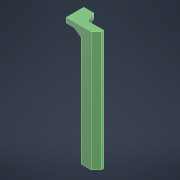
# Autodesk Inventor part: Vertical Beam Prototype
Saved by Autodesk Inventor 2022 (Build 260153000, 153)
## iProperties
Created: 2021-05-30
Part Number: Vertical Beam Prototype
Material: Generic
Document SubType Name: Modeling
Designer: sidsa
Density: 1 g/cm^3
Appearance: Smooth - Dark Forest Green
Author: sidsa
## iProperties of the stored document Vertical Beam Prototype_3DPrint.ipt
Created: 2021-05-30
Part Number: Vertical Beam Prototype_3DPrint
Material: Generic
Document SubType Name: Modeling
Designer: sidsa
Density: 1 g/cm^3
Appearance: Default
Author: sidsa
Autodesk Inventor part; units mm, degrees
ref_plane "YZ Plane" through (0, 0, 0) normal (1, 0, 0) x (0, 1, 0)
ref_plane "XZ Plane" through (0, 0, 0) normal (0, 1, 0) x (-1, 0, 0)
ref_plane "XY Plane" through (0, 0, 0) normal (0, 0, 1) x (1, 0, 0)
sketch "Sketch1" plane through (0, 0, 0) normal (0, 0, 1) x (1, 0, 0)
  line L0 (0, 0) -> (25.4, 0)
  line L1 (25.4, 0) -> (25.4, 152.4)
  line L2 (25.4, 152.4) -> (0, 152.4)
  line L3 (0, 152.4) -> (0, 0)
  line L4 (16.7357, 37.973) -> (20.3652, 31.6865)
  line L5 (20.3652, 31.6865) -> (16.7357, 25.4)
  line L6 (16.7357, 25.4) -> (9.4767, 25.4)
  line L7 (9.4767, 25.4) -> (5.8472, 31.6865)
  line L8 (5.8472, 31.6865) -> (9.4767, 37.973)
  line L9 (9.4767, 37.973) -> (16.7357, 37.973)
  line L10 (12.7, 0) -> (13.1062, 31.6865)
  dimension "d0" = 25.4
  dimension "d1" = 152.4
  dimension "d2" = 12.573
  dimension "d3" = 25.4
  constraints: 22 end point, 3 parallel, 1 horizontal, 1 midpoint, 1 perpendicular, 13 other
  measures "d0" distance of L1.end L2.end
  measures "d1" distance of L0.end L1.end
  measures "d2" distance between parallel lines of L6 L9
  measures "d3" distance between parallel lines of L0 L6
extrude "Extrusion1" add sketch "Sketch1" along normal blind 3.175
sketch "Sketch2" plane through (0, 0, 0) normal (0, 0, -1) x (-1, 0, 0)
  line L0 (-25.4, 0) -> (-25.4, 152.4) projected
  line L1 (0, 0) -> (-25.4, 0) projected
  line L2 (0, 152.4) -> (0, 0) projected
  line L3 (-25.4, 152.4) -> (0, 152.4) projected
  line L4 (-16.7357, 25.4) -> (-9.4767, 25.4) projected
  line L5 (-20.3652, 31.6865) -> (-16.7357, 25.4) projected
  line L6 (-16.7357, 37.973) -> (-20.3652, 31.6865) projected
  line L7 (-9.4767, 37.973) -> (-16.7357, 37.973) projected
  line L8 (-5.8472, 31.6865) -> (-9.4767, 37.973) projected
  line L9 (-9.4767, 25.4) -> (-5.8472, 31.6865) projected
extrude "Extrusion2" add sketch "Sketch2" along normal blind 3.175 and the other way blind 3.175 contours L5 L6 L7 L8 L9 L4
sketch "Sketch3" plane through (0, 0, 3.175) normal (0, 0, 1) x (1, 0, 0)
  line L0 (25.4, 0) -> (25.4, 152.4) projected
  line L1 (25.4, 152.4) -> (0, 152.4) projected
  line L2 (0, 152.4) -> (0, 0) projected
  line L3 (0, 0) -> (25.4, 0) projected
extrude "Extrusion3" add sketch "Sketch3" along normal blind 6.35
chamfer "Chamfer1" distance 6.35 angle 45 2 edges at (25.4, 76.2, 9.525) (0, 76.2, 9.525)
sketch "Sketch4" plane through (0, 152.4, 0) normal (0, 1, 0) x (1, 0, 0)
  line L0 (6.35, -9.525) -> (19.05, -9.525) projected
  line L1 (12.7, -9.525) -> (-12.7, -9.525)
  line L2 (-12.7, -9.525) -> (-12.7, 0)
  line L3 (-12.7, 0) -> (12.7, 0)
  line L4 (12.7, 0) -> (12.7, -9.525)
  line L5 (-12.7, 0) -> (0, 0)
  line L6 (0, 0) -> (0, 12.7)
  line L7 (0, 12.7) -> (-12.7, 12.7)
  line L8 (-12.7, 12.7) -> (-12.7, 0)
  line L9 (9.4767, 0) -> (5.8472, 0) projected
  line L10 (0, 12.7) -> (5.8472, 0)
  point P0 (0, 0)
  dimension "d15" = 25.4
  dimension "d16" = 12.7
  constraints: 18 end point, 4 parallel, 2 horizontal, 2 perpendicular, 1 midpoint
  measures "d15" distance of L1.start L1.end
  measures "d16" distance of L7.end L2.end
extrude "Extrusion4" add sketch "Sketch4" against normal blind 6.35
chamfer "Chamfer2" distance 6.35 angle 45 2 edges at (3.175, 146.05, 6.35) (0, 146.05, 1.5875)
chamfer "Chamfer3" distance 6.35 angle 45 2 edges at (-3.175, 146.05, 0) (2.9236, 146.05, 0)
body "Solid1"
